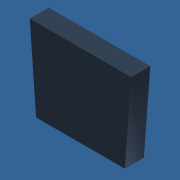
# Autodesk Inventor part: router keepout
Saved by Autodesk Inventor 2012 (Build 160160000, 160)
## iProperties
Created: 2012-03-25
Part Number: router keepout
Material: Default
Document SubType Name: Modeling
Designer: Edward
Density: 0.23658 g/cm^3
Mass: 283.495 g
Surface Area: 900.37 cm^2
Volume: 1198.3 cm^3
Author: Edward
Autodesk Inventor part; units mm, degrees
ref_plane "YZ Plane" through (0, 0, 0) normal (1, 0, 0) x (0, 1, 0)
ref_plane "XZ Plane" through (0, 0, 0) normal (0, 1, 0) x (-1, 0, 0)
ref_plane "XY Plane" through (0, 0, 0) normal (0, 0, 1) x (1, 0, 0)
sketch "Sketch1" plane through (0, 0, 0) normal (0, 0, 1) x (1, 0, 0)
  line L0 (-88.9, -82.55) -> (88.9, -82.55)
  line L1 (88.9, -82.55) -> (101.6, 82.55)
  line L2 (101.6, 82.55) -> (-101.6, 82.55)
  line L3 (-101.6, 82.55) -> (-88.9, -82.55)
  point P0 (0, 0)
  point P1 (0, 82.55)
  point P2 (-95.25, 0)
  dimension "d0" = 203.2
  dimension "d1" = 177.8
  dimension "d2" = 165.1
  constraints: 8 end point, 2 midpoint, 1 equal length, 1 horizontal, 1 horizontal alignment, 1 parallel, 1 vertical alignment
  measures "d0" distance of L1.end L2.end
  measures "d1" distance of L0.start L0.end
  measures "d2" distance between parallel lines of L0 L2
extrude "Extrusion1" add sketch "Sketch1" along normal blind 38.1
body "Solid1"
